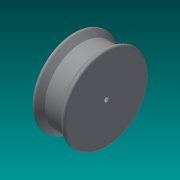
# Autodesk Inventor part: 22mm Spool
Saved by Autodesk Inventor 2013 (Build 170138000, 138)
## iProperties
Created: 2013-08-18
Part Number: 22mm Spool
Material: Generic
Document SubType Name: Modeling
Designer: Sawaiz
Density: 1 g/cm^3
Author: Sawaiz
Autodesk Inventor part; units mm, degrees
ref_plane "YZ Plane" through (0, 0, 0) normal (1, 0, 0) x (0, 1, 0)
ref_plane "XZ Plane" through (0, 0, 0) normal (0, 1, 0) x (-1, 0, 0)
ref_plane "XY Plane" through (0, 0, 0) normal (0, 0, 1) x (1, 0, 0)
sketch "Sketch1" plane through (0, 0, 0) normal (0, 0, 1) x (1, 0, 0)
  line L0 (1.5, -2) -> (1.5, 2)
  line L1 (-1.5, 2) -> (-1.5, -2)
  arc A0 (-1.5, -2) -> (1.5, -2) centre (0, 0) ccw
  arc A1 (1.5, 2) -> (-1.5, 2) centre (0, 0) ccw
  line L2 (-1.75, 2.1213) -> (-1.75, -2.1213)
  arc A2 (-1.75, -2.1213) -> (1.75, -2.1213) centre (0, 0) ccw
  line L3 (1.75, -2.1213) -> (1.75, 2.1213)
  arc A3 (1.75, 2.1213) -> (-1.75, 2.1213) centre (0, 0) ccw
  circle A4 centre (0, 0) radius 11
  dimension "d0" = 3
  dimension "d2" = 2.5
  dimension "d3" = 0.25
  dimension "d4" = 22
  constraints: 8 end point, 8 point on circle, 5 centre point, 2 coincident, 1 vertical, 4 other
  measures "d0" distance between parallel lines of L0 L1
  measures "d2" radius of A1
  measures "d3" distance between parallel lines of L1 L2
  measures "d4" diameter of A4
extrude "Extrusion1" add sketch "Sketch1" along normal blind 6 contours A4
sketch "Sketch2" plane through (0, 0, 6) normal (0, 0, 1) x (1, 0, 0)
  circle A0 centre (0, 0) radius 11 projected
extrude "Extrusion2" add sketch "Sketch2" along normal blind 2
sketch "Sketch3" plane through (0, 0, 8) normal (0, 0, 1) x (1, 0, 0)
  line L0 (0.5774, 0) -> (0.2887, -0.5)
  line L1 (0.2887, -0.5) -> (-0.2887, -0.5)
  line L2 (-0.2887, -0.5) -> (-0.5774, 0)
  line L3 (-0.5774, 0) -> (-0.2887, 0.5)
  line L4 (-0.2887, 0.5) -> (0.2887, 0.5)
  line L5 (0.2887, 0.5) -> (0.5774, 0)
  point P0 (0, 0)
  point P1 (0, 0)
  dimension "d24" = 1
  constraints: 12 end point, 1 coincident, 13 other
  measures "d24" distance between parallel lines of L1 L4
sketch "Sketch4" plane through (0, 0, 0) normal (1, 0, 0) x (0, 1, 0)
  line L0 (11, 8) -> (-11, 8) projected
  line L1 (-11, 0) -> (11, 0) projected
  line L2 (11, 8) -> (11, 0)
  line L3 (11, 0) -> (9, 2)
  line L4 (9, 2) -> (9, 6)
  line L5 (9, 6) -> (11, 8)
  line L6 (0, -1.6) -> (0, 9.6) projected
  point P0 (0, 0)
  dimension "d16" = 45
  dimension "d17" = 45
  dimension "d18" = 4
  constraints: 8 end point, 1 parallel, 1 perpendicular
  measures "d16" angle of L5 L2
  measures "d17" angle of L2 L3
  measures "d18" distance of L3.end L4.end
revolve "Revolution1" cut sketch "Sketch4" angle 360 about axis through (0, 0, -10) along (0, 0, 1) contours L2 L3 L4 L5
fillet "Fillet1" radius 0.5 2 edges at (0, -11, 0) (0, -11, 8)
extrude "Extrusion3" cut sketch "Sketch3" against normal through all
body "Solid1"
